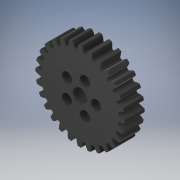
# Autodesk Inventor part: SE04
Saved by Autodesk Inventor 2017 SP1 (Build 210196100, 196)
## iProperties
Created: 2019-09-08
Part Number: SE04
Material: ABS Plastic
Document SubType Name: Modeling
Designer: Zach
Density: 1.06 g/cm^3
Appearance: Smooth - Black
Author: Zach
Autodesk Inventor part; units mm, degrees
(part 1 of 3)
ref_plane "YZ Plane" through (0, 0, 0) normal (1, 0, 0) x (0, 1, 0)
ref_plane "XZ Plane" through (0, 0, 0) normal (0, 1, 0) x (-1, 0, 0)
ref_plane "XY Plane" through (0, 0, 0) normal (0, 0, 1) x (1, 0, 0)
sketch "Sketch1" plane through (0, 0, 0) normal (0, 0, 1) x (1, 0, 0)
  arc A0 (-5.932911, 18.328081) -> (-5.539067, 18.99752) centre (-6.113075, 18.884647) ccw
  arc A1 (-5.932911, 18.328081) -> (-6.374085, 18.179357) centre (0.000012, -0.000078) ccw
  arc A2 (-7.092838, 18.47373) -> (-6.374085, 18.179357) centre (-6.567646, 18.731407) ccw
  spline S0 degree 3 poles (-9.030081, 20.608353) (-9.030081, 20.608353) (-9.030081, 20.608353) (-9.030081, 20.608353) (-9.030081, 20.608353) (-9.030081, 20.608353) (-9.030081, 20.608353) (-9.030081, 20.608353) (-9.030081, 20.608353) (-9.030081, 20.608353) (-9.030081, 20.608353) (-9.030081, 20.608353) (-9.030081, 20.608353) (-9.030081, 20.608353) (-9.030081, 20.608353) (-9.030029, 20.608313) (-9.023051, 20.602936) (-9.001036, 20.585861) (-8.989622, 20.576988) (-8.960537, 20.554257) (-8.942361, 20.539987) (-8.89306, 20.500976) (-8.860016, 20.474587) (-8.784661, 20.413566) (-8.741901, 20.378438) (-8.699366, 20.342893) knots 0 0 0 0 0.00003245 0.00003245 0.0000697 0.0000697 0.00012943 0.00012943 0.00021582 0.00021582 0.0003445 0.0003445 0.00053795 0.00053795 0.00077231 0.00077231 0.2100469 0.2100469 0.34914837 0.34914837 0.50737768 0.50737768 0.73605088 0.73605088 1 1 1 1
  spline S1 degree 3 poles (-8.699366, 20.342893) (-8.656399, 20.306988) (-8.538521, 20.206837) (-8.349354, 20.038244) (-8.135582, 19.833364) (-7.929716, 19.620545) (-7.73211, 19.400023) (-7.543618, 19.171666) (-7.362724, 18.937364) (-7.208648, 18.70567) (-7.128209, 18.545822) (-7.092838, 18.47373) knots 0 0 0 0 0.06771151 0.18704119 0.30636988 0.42569807 0.54502619 0.66435448 0.78368001 0.9029743 1 1 1 1
  arc A3 (-9.030081, 20.608353) -> (-10.023313, 20.143977) centre (0.000012, -0.000078) ccw
  arc A4 (-8.699366, 20.342893) -> (-10.031681, 19.719982) centre (0.000012, -0.000078) ccw
  arc A5 (-8.699366, 20.342893) -> (-10.031681, 19.719982) centre (0.000012, -0.000078) ccw
  spline S2 degree 3 poles (-10.031681, 19.719982) (-10.031681, 19.75177) (-10.031532, 19.78354) (-10.030954, 19.847219) (-10.030514, 19.879031) (-10.029214, 19.951703) (-10.028259, 19.991016) (-10.02666, 20.04753) (-10.026026, 20.067566) (-10.024905, 20.101012) (-10.02442, 20.114464) (-10.023579, 20.137231) (-10.023315, 20.14392) (-10.023313, 20.143977) (-10.023313, 20.143977) (-10.023313, 20.143977) (-10.023313, 20.143977) (-10.023313, 20.143977) (-10.023313, 20.143977) (-10.023313, 20.143977) (-10.023313, 20.143977) (-10.023313, 20.143977) (-10.023313, 20.143977) (-10.023313, 20.143977) (-10.023313, 20.143977) (-10.023313, 20.143977) (-10.023313, 20.143977) (-10.023313, 20.143977) knots 0 0 0 0 0.15149146 0.15149146 0.30980507 0.30980507 0.53062052 0.53062052 0.67593445 0.67593445 0.81687728 0.81687728 0.99922753 0.99922753 0.99946194 0.99946194 0.99965543 0.99965543 0.99978413 0.99978413 0.99987055 0.99987055 0.99993028 0.99993028 0.99996754 0.99996754 1 1 1 1
  spline S3 degree 3 poles (-9.627554, 17.288649) (-9.660192, 17.362018) (-9.73127, 17.526243) (-9.81026, 17.793043) (-9.874055, 18.082094) (-9.928415, 18.373163) (-9.970919, 18.666201) (-10.002215, 18.960638) (-10.022351, 19.256051) (-10.030418, 19.509315) (-10.031681, 19.663988) (-10.031681, 19.719982) knots 0 0 0 0 0.0970257 0.21631999 0.33564552 0.45497381 0.57430193 0.69363012 0.81295881 0.93228849 1 1 1 1
  spline S4 degree 3 poles (-5.392039, 21.457821) (-5.384966, 21.488811) (-5.377751, 21.519752) (-5.363018, 21.581705) (-5.355509, 21.612623) (-5.338071, 21.683183) (-5.328393, 21.721297) (-5.314258, 21.776039) (-5.309181, 21.795432) (-5.300646, 21.82779) (-5.29718, 21.840797) (-5.292456, 21.858461) (-5.290962, 21.864015) (-5.290178, 21.86693) (-5.289963, 21.867728) (-5.289748, 21.868526) (-5.289533, 21.869324) knots 0 0 0 0 0.15652291 0.15652291 0.32009454 0.32009454 0.54824388 0.54824388 0.69838409 0.69838409 0.84400801 0.84400801 0.96647827 0.96647827 0.96647827 1 1 1 1
  arc A6 (-4.217871, 22.101041) -> (-5.289533, 21.869324) centre (0.000012, -0.000078) ccw
  arc A7 (-3.954517, 21.768646) -> (-5.392039, 21.457821) centre (0.000012, -0.000078) ccw
  arc A8 (-3.954517, 21.768646) -> (-5.392039, 21.457821) centre (0.000012, -0.000078) ccw
  spline S5 degree 3 poles (-4.217871, 22.101041) (-4.217871, 22.101041) (-4.217871, 22.101041) (-4.217871, 22.101041) (-4.217871, 22.101041) (-4.217871, 22.101041) (-4.217871, 22.101041) (-4.217871, 22.101041) (-4.217871, 22.101041) (-4.217871, 22.101041) (-4.217871, 22.101041) (-4.217871, 22.101041) (-4.21787, 22.101041) (-4.21787, 22.101041) (-4.21787, 22.101041) (-4.217829, 22.100991) (-4.212222, 22.094196) (-4.194559, 22.07265) (-4.185405, 22.06146) (-4.162108, 22.032827) (-4.147562, 22.01487) (-4.108178, 21.965866) (-4.081835, 21.932786) (-4.021948, 21.856527) (-3.988076, 21.812764) (-3.954517, 21.768646) knots 0 0 0 0 0.00003245 0.00003245 0.0000697 0.0000697 0.00012943 0.00012943 0.00021582 0.00021582 0.0003445 0.0003445 0.00053795 0.00053795 0.00077231 0.00077231 0.21004691 0.21004691 0.34914837 0.34914837 0.50737768 0.50737768 0.73605088 0.73605088 1 1 1 1
  spline S6 degree 3 poles (-4.217871, 22.101041) (-4.217871, 22.101041) (-4.217871, 22.101041) (-4.217871, 22.101041) (-4.217871, 22.101041) (-4.217871, 22.101041) (-4.217871, 22.101041) (-4.217871, 22.101041) (-4.217871, 22.101041) (-4.217871, 22.101041) (-4.217871, 22.101041) (-4.217871, 22.101041) (-4.21787, 22.101041) (-4.21787, 22.101041) (-4.21787, 22.101041) (-4.217829, 22.100991) (-4.212222, 22.094196) (-4.194559, 22.07265) (-4.185405, 22.06146) (-4.162108, 22.032827) (-4.147562, 22.01487) (-4.108178, 21.965866) (-4.081835, 21.932786) (-4.021948, 21.856527) (-3.988076, 21.812764) (-3.954517, 21.768646) knots 0 0 0 0 0.00003245 0.00003245 0.0000697 0.0000697 0.00012943 0.00012943 0.00021582 0.00021582 0.0003445 0.0003445 0.00053795 0.00053795 0.00077231 0.00077231 0.21004691 0.21004691 0.34914837 0.34914837 0.50737768 0.50737768 0.73605088 0.73605088 1 1 1 1
  spline S7 degree 3 poles (-5.539067, 18.99752) (-5.554561, 19.076312) (-5.587313, 19.252235) (-5.604954, 19.529923) (-5.60283, 19.825922) (-5.591058, 20.12179) (-5.567289, 20.416939) (-5.532282, 20.710959) (-5.486177, 21.003445) (-5.437686, 21.252154) (-5.404499, 21.403231) (-5.392039, 21.457821) knots 0 0 0 0 0.0970257 0.21631999 0.33564552 0.45497381 0.57430193 0.69363012 0.81295881 0.93228849 1 1 1 1
  spline S8 degree 3 poles (-3.954517, 21.768646) (-3.920617, 21.72408) (-3.82798, 21.600209) (-3.681072, 21.39375) (-3.51825, 21.146438) (-3.364902, 20.893145) (-3.221321, 20.634181) (-3.088369, 20.369606) (-2.964148, 20.100926) (-2.865491, 19.840755) (-2.822639, 19.667016) (-2.804197, 19.588861) knots 0 0 0 0 0.06771151 0.18704119 0.30636988 0.42569807 0.54502619 0.66435448 0.78368001 0.9029743 1 1 1 1
  arc A9 (-2.804197, 19.588861) -> (-2.168968, 19.141931) centre (-2.234833, 19.723211) ccw
  arc A10 (-1.705761, 19.188755) -> (-2.168968, 19.141931) centre (0.000012, -0.000078) ccw
  arc A11 (-1.705761, 19.188755) -> (-1.172828, 19.753771) centre (-1.75756, 19.771457) ccw
  spline S9 degree 3 poles (3.252223, 19.519482) (3.27245, 19.597194) (3.319271, 19.769907) (3.423862, 20.027749) (3.554205, 20.293513) (3.693183, 20.554973) (3.842659, 20.81058) (4.001769, 21.060294) (4.170213, 21.303811) (4.321813, 21.50685) (4.417263, 21.628566) (4.452175, 21.672344) knots 0 0 0 0 0.0970257 0.21631999 0.33564552 0.45497381 0.57430193 0.69363012 0.81295881 0.93228849 1 1 1 1
  arc A12 (2.606923, 19.087221) -> (3.252223, 19.519482) centre (2.686086, 19.66684) ccw
  arc A13 (2.606923, 19.087221) -> (2.14491, 19.144644) centre (0.000012, -0.000078) ccw
  arc A14 (1.625059, 19.72172) -> (2.14491, 19.144644) centre (2.210044, 19.726007) ccw
  spline S10 degree 3 poles (0.988628, 22.102824) (1.011761, 22.051832) (1.074512, 21.910453) (1.171795, 21.67648) (1.275503, 21.399138) (1.368643, 21.118072) (1.450999, 20.833651) (1.521744, 20.546125) (1.583064, 20.256539) (1.621354, 19.980939) (1.624471, 19.80202) (1.625059, 19.72172) knots 0 0 0 0 0.06771151 0.18704119 0.30636988 0.42569807 0.54502619 0.66435448 0.78368001 0.9029743 1 1 1 1
  arc A15 (0.988628, 22.102824) -> (-0.482018, 22.119671) centre (0.000012, -0.000078) ccw
  spline S11 degree 3 poles (-1.172828, 19.753771) (-1.1704, 19.834036) (-1.163185, 20.012837) (-1.118592, 20.287488) (-1.050655, 20.575593) (-0.973342, 20.861423) (-0.884491, 21.143883) (-0.784937, 21.422741) (-0.674904, 21.697635) (-0.572285, 21.929318) (-0.506312, 22.069222) (-0.482018, 22.119671) knots 0 0 0 0 0.0970257 0.21631999 0.33564552 0.45497381 0.57430193 0.69363012 0.81295881 0.93228849 1 1 1 1
  spline S12 degree 3 poles (-0.482018, 22.119671) (-0.468226, 22.14831) (-0.454306, 22.17687) (-0.426157, 22.233991) (-0.411957, 22.262463) (-0.379255, 22.327374) (-0.361338, 22.362379) (-0.335376, 22.412603) (-0.326112, 22.430379) (-0.31059, 22.460027) (-0.304316, 22.471937) (-0.29578, 22.488106) (-0.293088, 22.493189) (-0.291674, 22.495857) (-0.291288, 22.496587) (-0.290901, 22.497317) (-0.290514, 22.498047) knots 0 0 0 0 0.15652267 0.15652267 0.32009406 0.32009406 0.54824306 0.54824306 0.69838305 0.69838305 0.84400675 0.84400675 0.96647984 0.96647984 0.96647984 1 1 1 1
  arc A16 (0.805842, 22.485487) -> (-0.290514, 22.498047) centre (0.000012, -0.000078) ccw
  arc A17 (0.805842, 22.485487) -> (-0.290514, 22.498047) centre (0.000012, -0.000078) ccw
  arc A18 (0.988628, 22.102824) -> (-0.482018, 22.119671) centre (0.000012, -0.000078) ccw
  spline S13 degree 3 poles (0.805842, 22.485487) (0.805842, 22.485487) (0.805842, 22.485487) (0.805842, 22.485487) (0.805842, 22.485487) (0.805842, 22.485487) (0.805842, 22.485487) (0.805842, 22.485487) (0.805842, 22.485487) (0.805842, 22.485487) (0.805842, 22.485487) (0.805842, 22.485487) (0.805842, 22.485487) (0.805842, 22.485487) (0.805842, 22.485487) (0.805872, 22.485428) (0.809826, 22.477557) (0.822252, 22.452621) (0.828686, 22.439674) (0.845028, 22.406575) (0.855213, 22.385832) (0.882705, 22.329293) (0.901027, 22.29118) (0.942443, 22.203506) (0.965727, 22.153304) (0.988628, 22.102824) knots 0 0 0 0 0.00003245 0.00003245 0.0000697 0.0000697 0.00012942 0.00012942 0.00021582 0.00021582 0.0003445 0.0003445 0.00053794 0.00053794 0.00077231 0.00077231 0.2100469 0.2100469 0.34914836 0.34914836 0.50737768 0.50737768 0.73605088 0.73605088 1 1 1 1
  spline S14 degree 3 poles (5.882199, 21.32867) (5.893406, 21.273809) (5.923123, 21.122012) (5.965904, 20.872258) (6.005297, 20.578791) (6.033559, 20.284047) (6.050561, 19.988431) (6.055552, 19.692372) (6.050895, 19.396401) (6.026898, 19.119191) (5.990123, 18.944064) (5.972829, 18.865647) knots 0 0 0 0 0.06771151 0.18704119 0.30636988 0.42569807 0.54502619 0.66435448 0.78368001 0.9029743 1 1 1 1
  spline S15 degree 3 poles (5.789147, 21.742413) (5.789147, 21.742413) (5.789147, 21.742413) (5.789147, 21.742413) (5.789147, 21.742413) (5.789147, 21.742413) (5.789147, 21.742413) (5.789147, 21.742413) (5.789147, 21.742413) (5.789147, 21.742413) (5.789147, 21.742413) (5.789147, 21.742413) (5.789147, 21.742413) (5.789147, 21.742413) (5.789147, 21.742413) (5.789163, 21.742349) (5.791266, 21.733795) (5.797832, 21.706719) (5.801224, 21.692665) (5.809791, 21.656759) (5.815105, 21.63427) (5.829327, 21.573031) (5.838708, 21.531797) (5.859577, 21.437105) (5.871106, 21.382981) (5.882199, 21.32867) knots 0 0 0 0 0.00003245 0.00003245 0.0000697 0.0000697 0.00012943 0.00012943 0.00021582 0.00021582 0.0003445 0.0003445 0.00053795 0.00053795 0.00077231 0.00077231 0.2100469 0.2100469 0.34914837 0.34914837 0.50737768 0.50737768 0.73605088 0.73605088 1 1 1 1
  arc A19 (5.789147, 21.742413) -> (4.723074, 21.99862) centre (0.000012, -0.000078) ccw
  arc A20 (5.882199, 21.32867) -> (4.452175, 21.672344) centre (0.000012, -0.000078) ccw
  arc A21 (5.882199, 21.32867) -> (4.452175, 21.672344) centre (0.000012, -0.000078) ccw
  spline S16 degree 3 poles (4.452175, 21.672344) (4.471994, 21.697196) (4.491919, 21.721943) (4.532074, 21.771368) (4.552253, 21.795966) (4.598579, 21.851973) (4.623836, 21.882113) (4.660323, 21.925301) (4.673311, 21.94057) (4.695041, 21.966021) (4.703808, 21.976236) (4.715728, 21.990101) (4.719484, 21.994457) (4.721455, 21.996743) (4.721995, 21.997369) (4.722534, 21.997994) (4.723074, 21.99862) knots 0 0 0 0 0.15652248 0.15652248 0.32009367 0.32009367 0.54824239 0.54824239 0.69838219 0.69838219 0.84400572 0.84400572 0.96648113 0.96648113 0.96648113 1 1 1 1
  arc A22 (5.972829, 18.865647) -> (6.351234, 18.187361) centre (6.5441, 18.739654) ccw
  arc A23 (6.788886, 18.02857) -> (6.351234, 18.187361) centre (0.000012, -0.000078) ccw
  arc A24 (6.788886, 18.02857) -> (7.514194, 18.306401) centre (6.995042, 18.576042) ccw
  spline S17 degree 3 poles (9.163118, 20.138272) (9.187969, 20.158097) (9.2129, 20.177795) (9.263044, 20.217057) (9.28819, 20.236554) (9.345815, 20.280861) (9.377145, 20.304633) (9.422326, 20.338629) (9.438385, 20.350629) (9.465232, 20.370612) (9.476052, 20.378623) (9.494375, 20.392164) (9.499769, 20.39613) (9.499815, 20.396164) (9.499815, 20.396164) (9.499815, 20.396164) (9.499815, 20.396164) (9.499815, 20.396164) (9.499815, 20.396164) (9.499815, 20.396164) (9.499815, 20.396164) (9.499815, 20.396164) (9.499815, 20.396164) (9.499815, 20.396164) (9.499815, 20.396164) (9.499815, 20.396164) (9.499815, 20.396164) (9.499815, 20.396164) knots 0 0 0 0 0.15149146 0.15149146 0.30980507 0.30980507 0.53062052 0.53062052 0.67593445 0.67593445 0.81687728 0.81687728 0.99922753 0.99922753 0.99946194 0.99946194 0.99965543 0.99965543 0.99978413 0.99978413 0.99987054 0.99987054 0.99993028 0.99993028 0.99996754 0.99996754 1 1 1 1
  spline S18 degree 3 poles (7.514194, 18.306401) (7.551207, 18.377664) (7.635286, 18.535627) (7.794629, 18.763731) (7.980843, 18.993828) (8.174517, 19.217807) (8.377123, 19.433744) (8.58781, 19.641792) (8.806219, 19.841721) (8.999198, 20.005936) (9.11934, 20.10336) (9.163118, 20.138272) knots 0 0 0 0 0.0970257 0.21631999 0.33564552 0.45497381 0.57430193 0.69363012 0.81295881 0.93228849 1 1 1 1
  arc A25 (10.482149, 19.909158) -> (9.499815, 20.396164) centre (0, 0) ccw
  arc A26 (10.480814, 19.485004) -> (9.163118, 20.138272) centre (0.000012, -0.000078) ccw
  arc A27 (10.480814, 19.485004) -> (9.163118, 20.138272) centre (0.000012, -0.000078) ccw
  spline S19 degree 3 poles (10.482149, 19.909158) (10.482162, 19.908332) (10.482175, 19.907507) (10.482188, 19.906682) (10.482245, 19.902983) (10.482366, 19.89518) (10.482674, 19.872419) (10.482855, 19.85796) (10.483218, 19.821042) (10.483395, 19.797929) (10.483635, 19.735049) (10.483607, 19.692754) (10.482884, 19.595775) (10.482082, 19.540432) (10.480814, 19.485004) knots 0 0 0 0 0.03353252 0.03353252 0.03353252 0.18383499 0.18383499 0.32755206 0.32755206 0.49103168 0.49103168 0.72729262 0.72729262 1 1 1 1
  spline S20 degree 3 poles (10.480814, 19.485004) (10.479531, 19.429025) (10.474726, 19.274421) (10.460858, 19.021409) (10.433961, 18.726535) (10.395928, 18.432891) (10.346723, 18.140904) (10.285709, 17.851156) (10.215309, 17.563643) (10.130228, 17.298722) (10.055407, 17.136169) (10.021097, 17.063567) knots 0 0 0 0 0.06771151 0.18704119 0.30636988 0.42569807 0.54502619 0.66435448 0.78368001 0.9029743 1 1 1 1
  arc A28 (10.021097, 17.063567) -> (10.239082, 16.318084) centre (10.550009, 16.813614) ccw
  arc A29 (10.630426, 16.065888) -> (10.239082, 16.318084) centre (0.000012, -0.000078) ccw
  arc A30 (10.630426, 16.065888) -> (11.399372, 16.175357) centre (10.953237, 16.553759) ccw
  spline S21 degree 3 poles (14.553877, 16.664275) (14.54017, 16.609984) (14.501082, 16.460326) (14.431262, 16.216743) (14.339423, 15.935247) (14.237002, 15.657429) (14.124057, 15.383712) (14.000098, 15.114806) (13.867486, 14.850166) (13.725588, 14.61082) (13.616471, 14.468992) (13.566865, 14.405845) knots 0 0 0 0 0.06771151 0.18704119 0.30636988 0.42569807 0.54502619 0.66435448 0.78368001 0.9029743 1 1 1 1
  spline S22 degree 3 poles (14.649556, 17.077418) (14.649556, 17.077418) (14.649556, 17.077418) (14.649556, 17.077418) (14.649556, 17.077418) (14.649556, 17.077418) (14.649556, 17.077418) (14.649556, 17.077418) (14.649556, 17.077418) (14.649556, 17.077418) (14.649556, 17.077418) (14.649556, 17.077418) (14.649556, 17.077418) (14.649556, 17.077418) (14.649556, 17.077418) (14.649542, 17.077354) (14.647726, 17.068734) (14.641893, 17.041491) (14.638852, 17.027357) (14.630991, 16.99129) (14.626021, 16.968722) (14.612264, 16.907377) (14.602826, 16.866156) (14.580542, 16.771787) (14.567446, 16.71802) (14.553877, 16.664275) knots 0 0 0 0 0.00003245 0.00003245 0.0000697 0.0000697 0.00012943 0.00012943 0.00021582 0.00021582 0.0003445 0.0003445 0.00053795 0.00053795 0.00077231 0.00077231 0.2100469 0.2100469 0.34914837 0.34914837 0.50737768 0.50737768 0.73605088 0.73605088 1 1 1 1
  arc A31 (14.553877, 16.664275) -> (13.414584, 17.594379) centre (0.000012, -0.000078) ccw
  arc A32 (14.553877, 16.664275) -> (13.414584, 17.594379) centre (0.000012, -0.000078) ccw
  arc A33 (14.649556, 17.077418) -> (13.800221, 17.770804) centre (0.000012, -0.000078) ccw
  spline S23 degree 3 poles (13.414584, 17.594379) (13.443223, 17.608171) (13.471912, 17.621821) (13.529535, 17.64893) (13.558389, 17.662336) (13.624427, 17.692696) (13.660261, 17.708893) (13.711873, 17.731972) (13.730199, 17.740095) (13.760819, 17.753596) (13.77315, 17.758996) (13.789906, 17.766316) (13.79518, 17.768611) (13.797948, 17.769816) (13.798706, 17.770145) (13.799463, 17.770475) (13.800221, 17.770804) knots 0 0 0 0 0.15652247 0.15652247 0.32009365 0.32009365 0.54824235 0.54824235 0.69838214 0.69838214 0.84400566 0.84400566 0.96648121 0.96648121 0.96648121 1 1 1 1
  spline S24 degree 3 poles (11.399372, 16.175357) (11.451315, 16.236597) (11.568436, 16.37189) (11.774542, 16.558818) (12.007288, 16.741709) (12.245947, 16.916976) (12.491523, 17.082415) (12.743223, 17.238364) (13.000644, 17.38468) (13.225326, 17.501836) (13.364135, 17.570084) (13.414584, 17.594379) knots 0 0 0 0 0.0970257 0.21631999 0.33564552 0.45497381 0.57430193 0.69363012 0.81295881 0.93228849 1 1 1 1
  spline S25 degree 3 poles (14.712939, 13.233209) (14.777206, 13.281355) (14.921497, 13.387194) (15.164031, 13.523572) (15.431639, 13.650087) (15.703314, 13.767854) (15.979547, 13.874499) (16.259638, 13.970529) (16.543164, 14.055895) (16.788282, 14.120117) (16.938797, 14.155766) (16.993387, 14.168226) knots 0 0 0 0 0.0970257 0.21631999 0.33564552 0.45497381 0.57430193 0.69363012 0.81295881 0.93228849 1 1 1 1
  arc A34 (13.938913, 13.297591) -> (14.712939, 13.233209) centre (14.362192, 13.701398) ccw
  arc A35 (13.938913, 13.297591) -> (13.6135, 13.630547) centre (0.000012, -0.000078) ccw
  arc A36 (13.566865, 14.405845) -> (13.6135, 13.630547) centre (14.026897, 14.044464) ccw
  arc A37 (16.065978, -10.630492) -> (16.318174, -10.239147) centre (0.000012, -0.000078) ccw
  arc A38 (17.063657, -10.021162) -> (16.318174, -10.239147) centre (16.813703, -10.550075) ccw
  spline S26 degree 3 poles (19.485094, -10.480879) (19.429115, -10.479597) (19.27451, -10.474791) (19.021498, -10.460924) (18.726624, -10.434027) (18.432981, -10.395993) (18.140994, -10.346788) (17.851246, -10.285774) (17.563733, -10.215375) (17.298812, -10.130294) (17.136259, -10.055473) (17.063657, -10.021162) knots 0 0 0 0 0.06771151 0.18704119 0.30636988 0.42569807 0.54502619 0.66435448 0.78368001 0.9029743 1 1 1 1
  spline S27 degree 3 poles (19.90917, -10.482227) (19.908344, -10.48224) (19.907519, -10.482252) (19.906694, -10.482265) (19.902996, -10.482322) (19.895194, -10.482443) (19.872438, -10.482751) (19.857981, -10.482931) (19.82107, -10.483293) (19.797962, -10.483469) (19.735093, -10.483708) (19.692805, -10.483678) (19.595844, -10.482953) (19.540511, -10.482149) (19.485094, -10.480879) knots 0 0 0 0 0.03353318 0.03353318 0.03353318 0.18383447 0.18383447 0.32755164 0.32755164 0.49103136 0.49103136 0.72729245 0.72729245 1 1 1 1
  arc A39 (19.90917, -10.482227) -> (20.396176, -9.499893) centre (0.000012, -0.000078) ccw
  arc A40 (19.485094, -10.480879) -> (20.138362, -9.163183) centre (0.000012, -0.000078) ccw
  arc A41 (19.485094, -10.480879) -> (20.138362, -9.163183) centre (0.000012, -0.000078) ccw
  spline S28 degree 3 poles (20.138362, -9.163183) (20.158181, -9.188036) (20.177873, -9.212968) (20.217124, -9.263114) (20.236615, -9.288261) (20.280908, -9.345888) (20.304673, -9.377219) (20.338659, -9.422401) (20.350655, -9.438461) (20.370632, -9.465309) (20.37864, -9.476129) (20.392177, -9.494453) (20.396142, -9.499847) (20.396176, -9.499893) (20.396176, -9.499893) (20.396176, -9.499893) (20.396176, -9.499893) (20.396176, -9.499893) (20.396176, -9.499893) (20.396176, -9.499893) (20.396176, -9.499893) (20.396176, -9.499893) (20.396176, -9.499893) (20.396176, -9.499893) (20.396176, -9.499893) (20.396176, -9.499893) (20.396176, -9.499893) (20.396176, -9.499893) knots 0 0 0 0 0.15149146 0.15149146 0.30980507 0.30980507 0.53062052 0.53062052 0.67593445 0.67593445 0.81687728 0.81687728 0.99922753 0.99922753 0.99946194 0.99946194 0.99965543 0.99965543 0.99978413 0.99978413 0.99987055 0.99987055 0.99993028 0.99993028 0.99996754 0.99996754 1 1 1 1
  spline S29 degree 3 poles (16.993387, 14.168226) (17.024378, 14.175299) (17.055385, 14.182223) (17.117595, 14.19583) (17.148708, 14.20248) (17.219847, 14.217384) (17.258387, 14.225201) (17.31384, 14.236217) (17.333515, 14.240057) (17.366371, 14.246407) (17.379595, 14.248927) (17.401977, 14.253173) (17.408557, 14.254405) (17.408614, 14.254416) (17.408614, 14.254416) (17.408614, 14.254416) (17.408614, 14.254416) (17.408614, 14.254416) (17.408614, 14.254416) (17.408614, 14.254416) (17.408614, 14.254416) (17.408614, 14.254416) (17.408614, 14.254416) (17.408614, 14.254416) (17.408614, 14.254416) (17.408614, 14.254416) (17.408614, 14.254416) (17.408614, 14.254416) knots 0 0 0 0 0.15149146 0.15149146 0.30980507 0.30980507 0.53062052 0.53062052 0.67593445 0.67593445 0.81687728 0.81687728 0.99922753 0.99922753 0.99946194 0.99946194 0.99965543 0.99965543 0.99978413 0.99978413 0.99987054 0.99987054 0.99993028 0.99993028 0.99996754 0.99996754 1 1 1 1
  arc A42 (17.897148, 13.007925) -> (16.993387, 14.168226) centre (0.000012, -0.000078) ccw
  arc A43 (17.897148, 13.007925) -> (16.993387, 14.168226) centre (0.000012, -0.000078) ccw
  arc A44 (18.082362, 13.389419) -> (17.408614, 14.254416) centre (0.000012, -0.000078) ccw
  spline S30 degree 3 poles (18.082362, 13.389419) (18.082362, 13.389419) (18.082362, 13.389419) (18.082362, 13.389419) (18.082362, 13.389419) (18.082362, 13.389419) (18.082362, 13.389419) (18.082362, 13.389419) (18.082362, 13.389419) (18.082362, 13.389419) (18.082362, 13.389419) (18.082362, 13.389419) (18.082362, 13.389419) (18.082362, 13.389419) (18.082361, 13.389419) (18.082334, 13.38936) (18.078645, 13.38136) (18.066896, 13.356098) (18.060786, 13.342995) (18.045097, 13.309582) (18.03523, 13.288686) (18.008167, 13.23194) (17.989793, 13.193852) (17.947069, 13.106808) (17.922337, 13.057303) (17.897148, 13.007925) knots 0 0 0 0 0.00003245 0.00003245 0.0000697 0.0000697 0.00012943 0.00012943 0.00021582 0.00021582 0.0003445 0.0003445 0.00053795 0.00053795 0.00077231 0.00077231 0.2100469 0.2100469 0.34914836 0.34914836 0.50737768 0.50737768 0.73605088 0.73605088 1 1 1 1
  arc A45 (16.432335, 11.025749) -> (16.30528, 10.259512) centre (16.800418, 10.571063) ccw
  arc A46 (16.548445, 9.862494) -> (16.30528, 10.259512) centre (0.000012, -0.000078) ccw
  spline S31 degree 3 poles (17.897148, 13.007925) (17.871704, 12.958046) (17.800294, 12.820837) (17.678023, 12.598898) (17.525848, 12.344896) (17.364174, 12.096835) (17.193153, 11.855112) (17.012465, 11.620532) (16.824289, 11.392037) (16.63269, 11.190266) (16.494749, 11.076275) (16.432335, 11.025749) knots 0 0 0 0 0.06771151 0.18704119 0.30636988 0.42569807 0.54502619 0.66435448 0.78368001 0.9029743 1 1 1 1
  arc A47 (16.548445, 9.862494) -> (17.288739, 9.627488) centre (17.050967, 10.161988) ccw
  spline S32 degree 3 poles (17.288739, 9.627488) (17.362108, 9.660126) (17.526333, 9.731205) (17.793133, 9.810194) (18.082183, 9.873989) (18.373252, 9.92835) (18.66629, 9.970853) (18.960728, 10.00215) (19.256141, 10.022285) (19.509404, 10.030353) (19.664078, 10.031615) (19.720072, 10.031615) knots 0 0 0 0 0.0970257 0.21631999 0.33564552 0.45497381 0.57430193 0.69363012 0.81295881 0.93228849 1 1 1 1
  arc A48 (18.082362, 13.389419) -> (17.408614, 14.254416) centre (0.000012, -0.000078) ccw
  spline S33 degree 3 poles (18.997609, 5.539001) (19.076402, 5.554495) (19.252325, 5.587248) (19.530013, 5.604888) (19.826012, 5.602764) (20.12188, 5.590993) (20.417028, 5.567223) (20.711048, 5.532217) (21.003535, 5.486112) (21.252244, 5.437621) (21.40332, 5.404433) (21.457911, 5.391973) knots 0 0 0 0 0.0970257 0.21631999 0.33564552 0.45497381 0.57430193 0.69363012 0.81295881 0.93228849 1 1 1 1
  arc A49 (18.32817, 5.932845) -> (18.997609, 5.539001) centre (18.884737, 6.113009) ccw
  arc A50 (18.32817, 5.932845) -> (18.179447, 6.374019) centre (0.000012, -0.000078) ccw
  arc A51 (18.47382, 7.092773) -> (18.179447, 6.374019) centre (18.731497, 6.56758) ccw
  spline S34 degree 3 poles (20.342983, 8.6993) (20.307077, 8.656333) (20.206926, 8.538455) (20.038334, 8.349288) (19.833454, 8.135517) (19.620634, 7.92965) (19.400113, 7.732044) (19.171756, 7.543552) (18.937454, 7.362659) (18.70576, 7.208582) (18.545911, 7.128143) (18.47382, 7.092773) knots 0 0 0 0 0.06771151 0.18704119 0.30636988 0.42569807 0.54502619 0.66435448 0.78368001 0.9029743 1 1 1 1
  spline S35 degree 3 poles (20.608443, 9.030015) (20.608443, 9.030015) (20.608443, 9.030015) (20.608443, 9.030015) (20.608443, 9.030015) (20.608443, 9.030015) (20.608443, 9.030015) (20.608443, 9.030015) (20.608443, 9.030015) (20.608443, 9.030015) (20.608443, 9.030015) (20.608443, 9.030015) (20.608443, 9.030015) (20.608443, 9.030015) (20.608443, 9.030015) (20.608402, 9.029963) (20.603026, 9.022986) (20.585951, 9.000971) (20.577078, 8.989556) (20.554347, 8.960471) (20.540077, 8.942295) (20.501066, 8.892994) (20.474677, 8.85995) (20.413655, 8.784595) (20.378527, 8.741835) (20.342983, 8.6993) knots 0 0 0 0 0.00003245 0.00003245 0.0000697 0.0000697 0.00012943 0.00012943 0.00021582 0.00021582 0.0003445 0.0003445 0.00053795 0.00053795 0.00077231 0.00077231 0.2100469 0.2100469 0.34914837 0.34914837 0.50737768 0.50737768 0.73605088 0.73605088 1 1 1 1
  spline S36 degree 3 poles (19.720072, 10.031615) (19.751859, 10.031615) (19.78363, 10.031466) (19.847308, 10.030888) (19.879121, 10.030448) (19.951793, 10.029148) (19.991105, 10.028194) (20.04762, 10.026594) (20.067656, 10.02596) (20.101102, 10.024839) (20.114554, 10.024354) (20.132827, 10.023679) (20.138574, 10.023459) (20.141591, 10.023343) (20.142416, 10.023311) (20.143242, 10.023279) (20.144067, 10.023247) knots 0 0 0 0 0.15652247 0.15652247 0.32009364 0.32009364 0.54824234 0.54824234 0.69838213 0.69838213 0.84400565 0.84400565 0.96648122 0.96648122 0.96648122 1 1 1 1
  arc A52 (20.342983, 8.6993) -> (19.720072, 10.031615) centre (0.000012, -0.000078) ccw
  arc A53 (20.342983, 8.6993) -> (19.720072, 10.031615) centre (0.000012, -0.000078) ccw
  arc A54 (20.608443, 9.030015) -> (20.144067, 10.023247) centre (0.000012, -0.000078) ccw
  arc A55 (21.742503, -5.789213) -> (21.998709, -4.723139) centre (0.000012, -0.000078) ccw
  arc A56 (21.32876, -5.882265) -> (21.672434, -4.452241) centre (0.000012, -0.000078) ccw
  arc A57 (21.32876, -5.882265) -> (21.672434, -4.452241) centre (0.000012, -0.000078) ccw
  spline S37 degree 3 poles (21.742503, -5.789213) (21.741701, -5.789409) (21.7409, -5.789605) (21.740098, -5.789801) (21.736506, -5.79068) (21.728926, -5.792534) (21.706809, -5.797897) (21.692755, -5.80129) (21.656849, -5.809856) (21.63436, -5.81517) (21.573121, -5.829392) (21.531887, -5.838774) (21.437195, -5.859642) (21.38307, -5.871172) (21.32876, -5.882265) knots 0 0 0 0 0.03353253 0.03353253 0.03353253 0.18383498 0.18383498 0.32755205 0.32755205 0.49103167 0.49103167 0.72729262 0.72729262 1 1 1 1
  arc A58 (18.865736, -5.972895) -> (18.187451, -6.3513) centre (18.739744, -6.544166) ccw
  arc A59 (18.02866, -6.788951) -> (18.187451, -6.3513) centre (0.000012, -0.000078) ccw
  arc A60 (18.02866, -6.788951) -> (18.306491, -7.514259) centre (18.576131, -6.995107) ccw
  spline S38 degree 3 poles (18.306491, -7.514259) (18.377753, -7.551272) (18.535717, -7.635352) (18.763821, -7.794695) (18.993918, -7.980909) (19.217897, -8.174582) (19.433834, -8.377188) (19.641881, -8.587876) (19.841811, -8.806284) (20.006025, -8.999264) (20.10345, -9.119405) (20.138362, -9.163183) knots 0 0 0 0 0.0970257 0.21631999 0.33564552 0.45497381 0.57430193 0.69363012 0.81295881 0.93228849 1 1 1 1
  spline S39 degree 3 poles (21.32876, -5.882265) (21.273899, -5.893471) (21.122102, -5.923189) (20.872347, -5.96597) (20.578881, -6.005363) (20.284137, -6.033625) (19.988521, -6.050627) (19.692461, -6.055617) (19.396491, -6.05096) (19.11928, -6.026963) (18.944153, -5.990189) (18.865736, -5.972895) knots 0 0 0 0 0.06771151 0.18704119 0.30636988 0.42569807 0.54502619 0.66435448 0.78368001 0.9029743 1 1 1 1
  spline S40 degree 3 poles (21.457911, 5.391973) (21.488901, 5.3849) (21.519842, 5.377685) (21.581795, 5.362952) (21.612712, 5.355444) (21.683273, 5.338006) (21.721387, 5.328327) (21.776129, 5.314192) (21.795521, 5.309116) (21.827879, 5.300581) (21.840887, 5.297114) (21.862895, 5.291228) (21.869358, 5.289483) (21.869413, 5.289468) (21.869413, 5.289468) (21.869413, 5.289468) (21.869413, 5.289468) (21.869413, 5.289468) (21.869413, 5.289468) (21.869413, 5.289468) (21.869413, 5.289468) (21.869413, 5.289468) (21.869413, 5.289468) (21.869413, 5.289468) (21.869413, 5.289468) (21.869413, 5.289468) (21.869413, 5.289468) (21.869413, 5.289468) knots 0 0 0 0 0.15149146 0.15149146 0.30980507 0.30980507 0.53062052 0.53062052 0.67593445 0.67593445 0.81687728 0.81687728 0.99922753 0.99922753 0.99946194 0.99946194 0.99965543 0.99965543 0.99978414 0.99978414 0.99987055 0.99987055 0.99993029 0.99993029 0.99996754 0.99996754 1 1 1 1
  arc A61 (21.768736, 3.954452) -> (21.457911, 5.391973) centre (0.000012, -0.000078) ccw
  arc A62 (21.768736, 3.954452) -> (21.457911, 5.391973) centre (0.000012, -0.000078) ccw
  arc A63 (22.101131, 4.217805) -> (21.869413, 5.289468) centre (0.000012, -0.000078) ccw
  spline S41 degree 3 poles (22.101131, 4.217805) (22.101131, 4.217805) (22.101131, 4.217805) (22.101131, 4.217805) (22.101131, 4.217805) (22.101131, 4.217805) (22.101131, 4.217805) (22.101131, 4.217805) (22.101131, 4.217805) (22.101131, 4.217805) (22.101131, 4.217805) (22.101131, 4.217805) (22.101131, 4.217805) (22.101131, 4.217805) (22.101131, 4.217805) (22.10108, 4.217763) (22.094286, 4.212157) (22.07274, 4.194493) (22.06155, 4.185339) (22.032917, 4.162042) (22.01496, 4.147497) (21.965956, 4.108112) (21.932876, 4.081769) (21.856616, 4.021882) (21.812854, 3.988011) (21.768736, 3.954452) knots 0 0 0 0 0.00003245 0.00003245 0.0000697 0.0000697 0.00012943 0.00012943 0.00021582 0.00021582 0.0003445 0.0003445 0.00053795 0.00053795 0.00077231 0.00077231 0.21004691 0.21004691 0.34914837 0.34914837 0.50737768 0.50737768 0.73605088 0.73605088 1 1 1 1
  spline S42 degree 3 poles (21.768736, 3.954452) (21.724169, 3.920552) (21.600299, 3.827915) (21.39384, 3.681006) (21.146528, 3.518184) (20.893235, 3.364836) (20.634271, 3.221255) (20.369696, 3.088303) (20.101015, 2.964082) (19.840845, 2.865426) (19.667105, 2.822573) (19.588951, 2.804131) knots 0 0 0 0 0.06771151 0.18704119 0.30636988 0.42569807 0.54502619 0.66435448 0.78368001 0.9029743 1 1 1 1
  arc A64 (19.188845, 1.705696) -> (19.14202, 2.168903) centre (0.000012, -0.000078) ccw
  arc A65 (19.188845, 1.705696) -> (19.753861, 1.172762) centre (19.771547, 1.757495) ccw
  spline S43 degree 3 poles (19.753861, 1.172762) (19.834125, 1.170334) (20.012926, 1.163119) (20.287577, 1.118526) (20.575682, 1.050589) (20.861513, 0.973276) (21.143972, 0.884426) (21.422831, 0.784871) (21.697725, 0.674838) (21.929408, 0.57222) (22.069312, 0.506247) (22.11976, 0.481952) knots 0 0 0 0 0.0970257 0.21631999 0.33564552 0.45497381 0.57430193 0.69363012 0.81295881 0.93228849 1 1 1 1
  arc A66 (19.588951, 2.804131) -> (19.14202, 2.168903) centre (19.723301, 2.234768) ccw
  spline S44 degree 3 poles (19.519572, -3.252288) (19.597284, -3.272516) (19.769996, -3.319337) (20.027838, -3.423928) (20.293603, -3.554271) (20.555063, -3.693249) (20.81067, -3.842724) (21.060383, -4.001835) (21.303901, -4.170279) (21.50694, -4.321878) (21.628656, -4.417329) (21.672434, -4.452241) knots 0 0 0 0 0.0970257 0.21631999 0.33564552 0.45497381 0.57430193 0.69363012 0.81295881 0.93228849 1 1 1 1
  arc A67 (19.087311, -2.606988) -> (19.519572, -3.252288) centre (19.66693, -2.686152) ccw
  arc A68 (19.087311, -2.606988) -> (19.144734, -2.144976) centre (0.000012, -0.000078) ccw
  arc A69 (19.72181, -1.625125) -> (19.144734, -2.144976) centre (19.726097, -2.210109) ccw
  spline S45 degree 3 poles (22.102914, -0.988693) (22.051921, -1.011826) (21.910543, -1.074577) (21.67657, -1.171861) (21.399228, -1.275568) (21.118162, -1.368709) (20.833741, -1.451065) (20.546215, -1.52181) (20.256629, -1.58313) (19.981028, -1.621419) (19.802109, -1.624537) (19.72181, -1.625125) knots 0 0 0 0 0.06771151 0.18704119 0.30636988 0.42569807 0.54502619 0.66435448 0.78368001 0.9029743 1 1 1 1
  spline S46 degree 3 poles (22.485577, -0.805908) (22.484839, -0.806278) (22.484101, -0.806647) (22.483364, -0.807017) (22.480056, -0.808673) (22.47308, -0.812167) (22.45271, -0.822317) (22.439764, -0.828752) (22.406664, -0.845094) (22.385921, -0.855278) (22.329382, -0.882771) (22.29127, -0.901093) (22.203596, -0.942509) (22.153394, -0.965793) (22.102914, -0.988693) knots 0 0 0 0 0.03353406 0.03353406 0.03353406 0.18383379 0.18383379 0.32755107 0.32755107 0.49103093 0.49103093 0.72729222 0.72729222 1 1 1 1
  arc A70 (22.485577, -0.805908) -> (22.498136, 0.290448) centre (0.000012, -0.000078) ccw
  arc A71 (22.102914, -0.988693) -> (22.11976, 0.481952) centre (0.000012, -0.000078) ccw
  arc A72 (22.102914, -0.988693) -> (22.11976, 0.481952) centre (0.000012, -0.000078) ccw
  spline S47 degree 3 poles (22.11976, 0.481952) (22.1484, 0.46816) (22.17696, 0.454241) (22.234081, 0.426091) (22.262552, 0.411891) (22.327463, 0.379189) (22.362469, 0.361272) (22.412692, 0.335311) (22.430469, 0.326046) (22.460116, 0.310525) (22.472026, 0.304251) (22.488196, 0.295714) (22.493279, 0.293022) (22.495946, 0.291609) (22.496676, 0.291222) (22.497406, 0.290835) (22.498136, 0.290448) knots 0 0 0 0 0.15652292 0.15652292 0.32009458 0.32009458 0.54824394 0.54824394 0.69838416 0.69838416 0.8440081 0.8440081 0.96647816 0.96647816 0.96647816 1 1 1 1
  spline S48 degree 3 poles (21.672434, -4.452241) (21.697286, -4.47206) (21.722033, -4.491985) (21.771458, -4.532139) (21.796056, -4.552319) (21.852062, -4.598645) (21.882203, -4.623902) (21.925391, -4.660389) (21.94066, -4.673377) (21.96611, -4.695106) (21.976325, -4.703873) (21.99019, -4.715794) (21.994547, -4.71955) (21.996833, -4.721521) (21.997458, -4.72206) (21.998084, -4.7226) (21.998709, -4.723139) knots 0 0 0 0 0.1565225 0.1565225 0.32009372 0.32009372 0.54824247 0.54824247 0.69838228 0.69838228 0.84400583 0.84400583 0.96648099 0.96648099 0.96648099 1 1 1 1
  spline S49 degree 3 poles (-21.328736, 5.88211) (-21.273875, 5.893316) (-21.122078, 5.923034) (-20.872323, 5.965815) (-20.578857, 6.005207) (-20.284113, 6.033469) (-19.988497, 6.050471) (-19.692437, 6.055462) (-19.396467, 6.050805) (-19.119256, 6.026808) (-18.944129, 5.990034) (-18.865712, 5.972739) knots 0 0 0 0 0.06771151 0.18704119 0.30636988 0.42569807 0.54502619 0.66435448 0.78368001 0.9029743 1 1 1 1
  spline S50 degree 3 poles (-21.742479, 5.789058) (-21.741677, 5.789254) (-21.740876, 5.78945) (-21.740074, 5.789646) (-21.736482, 5.790525) (-21.728902, 5.792379) (-21.706785, 5.797742) (-21.692731, 5.801135) (-21.656825, 5.809701) (-21.634336, 5.815015) (-21.573097, 5.829237) (-21.531863, 5.838619) (-21.437171, 5.859487) (-21.383046, 5.871016) (-21.328736, 5.88211) knots 0 0 0 0 0.03353302 0.03353302 0.03353302 0.1838346 0.1838346 0.32755174 0.32755174 0.49103143 0.49103143 0.72729249 0.72729249 1 1 1 1
  arc A73 (-21.328736, 5.88211) -> (-21.67241, 4.452085) centre (0.000012, -0.000078) ccw
  arc A74 (-21.742479, 5.789058) -> (-21.998685, 4.722984) centre (0.000012, -0.000078) ccw
  spline S51 degree 3 poles (-21.67241, 4.452085) (-21.697262, 4.471904) (-21.722008, 4.49183) (-21.771434, 4.531984) (-21.796032, 4.552163) (-21.852038, 4.59849) (-21.882179, 4.623747) (-21.925366, 4.660234) (-21.940636, 4.673221) (-21.966086, 4.694951) (-21.976301, 4.703718) (-21.990166, 4.715638) (-21.994522, 4.719394) (-21.996808, 4.721365) (-21.997434, 4.721905) (-21.99806, 4.722444) (-21.998685, 4.722984) knots 0 0 0 0 0.15652271 0.15652271 0.32009414 0.32009414 0.54824319 0.54824319 0.69838321 0.69838321 0.84400695 0.84400695 0.9664796 0.9664796 0.9664796 1 1 1 1
  arc A75 (-21.328736, 5.88211) -> (-21.67241, 4.452085) centre (0.000012, -0.000078) ccw
  arc A76 (-19.588926, -2.804287) -> (-19.141996, -2.169058) centre (-19.723277, -2.234923) ccw
  spline S52 degree 3 poles (-21.768711, -3.954607) (-21.724145, -3.920707) (-21.600275, -3.82807) (-21.393816, -3.681161) (-21.146504, -3.51834) (-20.893211, -3.364992) (-20.634247, -3.22141) (-20.369672, -3.088459) (-20.100991, -2.964238) (-19.840821, -2.865581) (-19.667081, -2.822729) (-19.588926, -2.804287) knots 0 0 0 0 0.06771151 0.18704119 0.30636988 0.42569807 0.54502619 0.66435448 0.78368001 0.9029743 1 1 1 1
  spline S53 degree 3 poles (-22.101107, -4.21796) (-22.101107, -4.21796) (-22.101107, -4.21796) (-22.101107, -4.21796) (-22.101107, -4.21796) (-22.101107, -4.21796) (-22.101107, -4.21796) (-22.101107, -4.21796) (-22.101107, -4.21796) (-22.101107, -4.21796) (-22.101107, -4.21796) (-22.101107, -4.21796) (-22.101107, -4.21796) (-22.101107, -4.21796) (-22.101107, -4.21796) (-22.101056, -4.217918) (-22.094262, -4.212312) (-22.072716, -4.194649) (-22.061525, -4.185494) (-22.032893, -4.162197) (-22.014936, -4.147652) (-21.965932, -4.108268) (-21.932852, -4.081924) (-21.856592, -4.022037) (-21.81283, -3.988166) (-21.768711, -3.954607) knots 0 0 0 0 0.00003245 0.00003245 0.0000697 0.0000697 0.00012942 0.00012942 0.00021582 0.00021582 0.0003445 0.0003445 0.00053795 0.00053795 0.00077231 0.00077231 0.2100469 0.2100469 0.34914836 0.34914836 0.50737768 0.50737768 0.73605088 0.73605088 1 1 1 1
  arc A77 (-22.101107, -4.21796) -> (-21.869389, -5.289623) centre (0.000012, -0.000078) ccw
  arc A78 (-21.768711, -3.954607) -> (-21.457887, -5.392129) centre (0.000012, -0.000078) ccw
  arc A79 (-21.768711, -3.954607) -> (-21.457887, -5.392129) centre (0.000012, -0.000078) ccw
  spline S54 degree 3 poles (-21.457887, -5.392129) (-21.488877, -5.385055) (-21.519818, -5.37784) (-21.581771, -5.363108) (-21.612688, -5.355599) (-21.683249, -5.338161) (-21.721363, -5.328483) (-21.776105, -5.314348) (-21.795497, -5.309271) (-21.827855, -5.300736) (-21.840862, -5.297269) (-21.862871, -5.291383) (-21.869334, -5.289638) (-21.869389, -5.289623) (-21.869389, -5.289623) (-21.869389, -5.289623) (-21.869389, -5.289623) (-21.869389, -5.289623) (-21.869389, -5.289623) (-21.869389, -5.289623) (-21.869389, -5.289623) (-21.869389, -5.289623) (-21.869389, -5.289623) (-21.869389, -5.289623) (-21.869389, -5.289623) (-21.869389, -5.289623) (-21.869389, -5.289623) (-21.869389, -5.289623) knots 0 0 0 0 0.15149146 0.15149146 0.30980507 0.30980507 0.53062052 0.53062052 0.67593445 0.67593445 0.81687728 0.81687728 0.99922753 0.99922753 0.99946194 0.99946194 0.99965543 0.99965543 0.99978414 0.99978414 0.99987055 0.99987055 0.99993029 0.99993029 0.99996754 0.99996754 1 1 1 1
  spline S55 degree 3 poles (-10.48079, -19.48516) (-10.479507, -19.42918) (-10.474702, -19.274576) (-10.460834, -19.021564) (-10.433937, -18.72669) (-10.395904, -18.433046) (-10.346699, -18.141059) (-10.285685, -17.851312) (-10.215285, -17.563798) (-10.130204, -17.298878) (-10.055383, -17.136325) (-10.021072, -17.063722) knots 0 0 0 0 0.06771151 0.18704119 0.30636988 0.42569807 0.54502619 0.66435448 0.78368001 0.9029743 1 1 1 1
  spline S56 degree 3 poles (-10.482137, -19.909235) (-10.482137, -19.909235) (-10.482137, -19.909235) (-10.482137, -19.909235) (-10.482137, -19.909235) (-10.482137, -19.909235) (-10.482137, -19.909235) (-10.482137, -19.909235) (-10.482137, -19.909235) (-10.482137, -19.909235) (-10.482137, -19.909235) (-10.482137, -19.909235) (-10.482137, -19.909235) (-10.482137, -19.909235) (-10.482137, -19.909235) (-10.482138, -19.909169) (-10.482285, -19.900362) (-10.482661, -19.872503) (-10.482841, -19.858047) (-10.483203, -19.821135) (-10.483379, -19.798027) (-10.483618, -19.735159) (-10.483589, -19.692871) (-10.482863, -19.59591) (-10.482059, -19.540577) (-10.48079, -19.48516) knots 0 0 0 0 0.00003245 0.00003245 0.0000697 0.0000697 0.00012943 0.00012943 0.00021582 0.00021582 0.0003445 0.0003445 0.00053795 0.00053795 0.00077231 0.00077231 0.2100469 0.2100469 0.34914837 0.34914837 0.50737768 0.50737768 0.73605088 0.73605088 1 1 1 1
  arc A80 (-10.48079, -19.48516) -> (-9.163094, -20.138427) centre (0.000012, -0.000078) ccw
  arc A81 (-10.48079, -19.48516) -> (-9.163094, -20.138427) centre (0.000012, -0.000078) ccw
  arc A82 (-10.482137, -19.909235) -> (-9.499803, -20.396242) centre (0.000012, -0.000078) ccw
  spline S57 degree 3 poles (-9.163094, -20.138427) (-9.187946, -20.158246) (-9.212878, -20.177938) (-9.263024, -20.21719) (-9.288171, -20.23668) (-9.345798, -20.280974) (-9.377129, -20.304739) (-9.422311, -20.338724) (-9.438371, -20.350721) (-9.465219, -20.370698) (-9.476039, -20.378706) (-9.494363, -20.392243) (-9.499757, -20.396208) (-9.499803, -20.396242) (-9.499803, -20.396242) (-9.499803, -20.396242) (-9.499803, -20.396242) (-9.499803, -20.396242) (-9.499803, -20.396242) (-9.499803, -20.396242) (-9.499803, -20.396242) (-9.499803, -20.396242) (-9.499803, -20.396242) (-9.499803, -20.396242) (-9.499803, -20.396242) (-9.499803, -20.396242) (-9.499803, -20.396242) (-9.499803, -20.396242) knots 0 0 0 0 0.15149146 0.15149146 0.30980507 0.30980507 0.53062052 0.53062052 0.67593445 0.67593445 0.81687728 0.81687728 0.99922753 0.99922753 0.99946194 0.99946194 0.99965543 0.99965543 0.99978413 0.99978413 0.99987055 0.99987055 0.99993028 0.99993028 0.99996754 0.99996754 1 1 1 1
  spline S58 degree 3 poles (-7.51417, -18.306557) (-7.551183, -18.377819) (-7.635262, -18.535783) (-7.794605, -18.763886) (-7.980819, -18.993983) (-8.174493, -19.217963) (-8.377098, -19.433899) (-8.587786, -19.641947) (-8.806195, -19.841876) (-8.999174, -20.006091) (-9.119316, -20.103515) (-9.163094, -20.138427) knots 0 0 0 0 0.0970257 0.21631999 0.33564552 0.45497381 0.57430193 0.69363012 0.81295881 0.93228849 1 1 1 1
  spline S59 degree 3 poles (-0.805818, -22.485643) (-0.806188, -22.484905) (-0.806557, -22.484167) (-0.806927, -22.483429) (-0.808583, -22.480122) (-0.812077, -22.473145) (-0.822228, -22.452776) (-0.828662, -22.439829) (-0.845004, -22.40673) (-0.855189, -22.385987) (-0.882681, -22.329448) (-0.901003, -22.291335) (-0.942419, -22.203661) (-0.965703, -22.153459) (-0.988604, -22.102979) knots 0 0 0 0 0.03353315 0.03353315 0.03353315 0.1838345 0.1838345 0.32755165 0.32755165 0.49103137 0.49103137 0.72729246 0.72729246 1 1 1 1
  arc A83 (-0.988604, -22.102979) -> (0.482042, -22.119826) centre (0.000012, -0.000078) ccw
  arc A84 (-0.988604, -22.102979) -> (0.482042, -22.119826) centre (0.000012, -0.000078) ccw
  arc A85 (-0.805818, -22.485643) -> (0.290538, -22.498202) centre (0.000012, -0.000078) ccw
  spline S60 degree 3 poles (0.482042, -22.119826) (0.46825, -22.148465) (0.45433, -22.177025) (0.426181, -22.234147) (0.411981, -22.262618) (0.379279, -22.327529) (0.361362, -22.362534) (0.3354, -22.412758) (0.326136, -22.430535) (0.310614, -22.460182) (0.30434, -22.472092) (0.293705, -22.492238) (0.290565, -22.498151) (0.290538, -22.498202) (0.290538, -22.498202) (0.290538, -22.498202) (0.290538, -22.498202) (0.290538, -22.498202) (0.290538, -22.498202) (0.290538, -22.498202) (0.290538, -22.498202) (0.290538, -22.498202) (0.290538, -22.498202) (0.290538, -22.498202) (0.290538, -22.498202) (0.290538, -22.498202) (0.290538, -22.498202) (0.290538, -22.498202) knots 0 0 0 0 0.15149146 0.15149146 0.30980507 0.30980507 0.53062052 0.53062052 0.67593445 0.67593445 0.81687728 0.81687728 0.99922753 0.99922753 0.99946194 0.99946194 0.99965543 0.99965543 0.99978413 0.99978413 0.99987055 0.99987055 0.99993028 0.99993028 0.99996754 0.99996754 1 1 1 1
  spline S61 degree 3 poles (17.594468, -13.414649) (17.60826, -13.443289) (17.621911, -13.471978) (17.649019, -13.529601) (17.662426, -13.558454) (17.692786, -13.624493) (17.708983, -13.660326) (17.732062, -13.711938) (17.740184, -13.730265) (17.753686, -13.760885) (17.759086, -13.773216) (17.766406, -13.789972) (17.768701, -13.795246) (17.769905, -13.798013) (17.770235, -13.798771) (17.770564, -13.799529) (17.770894, -13.800286) knots 0 0 0 0 0.15652274 0.15652274 0.32009419 0.32009419 0.54824328 0.54824328 0.69838332 0.69838332 0.84400708 0.84400708 0.96647943 0.96647943 0.96647943 1 1 1 1
  spline S62 degree 3 poles (16.175447, -11.399438) (16.236686, -11.45138) (16.37198, -11.568502) (16.558907, -11.774608) (16.741799, -12.007354) (16.917066, -12.246012) (17.082505, -12.491589) (17.238454, -12.743289) (17.38477, -13.00071) (17.501926, -13.225392) (17.570173, -13.3642) (17.594468, -13.414649) knots 0 0 0 0 0.0970257 0.21631999 0.33564552 0.45497381 0.57430193 0.69363012 0.81295881 0.93228849 1 1 1 1
  arc A86 (17.077508, -14.649622) -> (17.770894, -13.800286) centre (0.000012, -0.000078) ccw
  arc A87 (16.664365, -14.553942) -> (17.594468, -13.414649) centre (0.000012, -0.000078) ccw
  arc A88 (16.664365, -14.553942) -> (17.594468, -13.414649) centre (0.000012, -0.000078) ccw
  spline S63 degree 3 poles (17.077508, -14.649622) (17.077508, -14.649622) (17.077508, -14.649622) (17.077508, -14.649622) (17.077508, -14.649622) (17.077508, -14.649622) (17.077508, -14.649622) (17.077508, -14.649622) (17.077508, -14.649622) (17.077508, -14.649622) (17.077508, -14.649622) (17.077508, -14.649622) (17.077508, -14.649622) (17.077508, -14.649622) (17.077508, -14.649622) (17.077443, -14.649608) (17.068824, -14.647791) (17.04158, -14.641959) (17.027446, -14.638918) (16.99138, -14.631057) (16.968812, -14.626087) (16.907466, -14.61233) (16.866245, -14.602892) (16.771877, -14.580608) (16.71811, -14.567512) (16.664365, -14.553942) knots 0 0 0 0 0.00003245 0.00003245 0.0000697 0.0000697 0.00012943 0.00012943 0.00021582 0.00021582 0.0003445 0.0003445 0.00053795 0.00053795 0.00077231 0.00077231 0.2100469 0.2100469 0.34914836 0.34914836 0.50737768 0.50737768 0.73605088 0.73605088 1 1 1 1
  spline S64 degree 3 poles (16.664365, -14.553942) (16.610074, -14.540235) (16.460416, -14.501148) (16.216833, -14.431328) (15.935337, -14.339489) (15.657519, -14.237067) (15.383802, -14.124123) (15.114896, -14.000164) (14.850256, -13.867551) (14.61091, -13.725654) (14.469082, -13.616536) (14.405934, -13.566931) knots 0 0 0 0 0.06771151 0.18704119 0.30636988 0.42569807 0.54502619 0.66435448 0.78368001 0.9029743 1 1 1 1
  arc A89 (14.405934, -13.566931) -> (13.630636, -13.613565) centre (14.044554, -14.026962) ccw
  arc A90 (13.297681, -13.938979) -> (13.630636, -13.613565) centre (0.000012, -0.000078) ccw
  arc A91 (13.297681, -13.938979) -> (13.233298, -14.713005) centre (13.701488, -14.362258) ccw
  spline S65 degree 3 poles (14.168315, -16.993453) (14.175389, -17.024443) (14.182313, -17.05545) (14.19592, -17.117661) (14.202569, -17.148774) (14.217473, -17.219913) (14.225291, -17.258452) (14.236307, -17.313906) (14.240147, -17.33358) (14.246497, -17.366437) (14.249017, -17.37966) (14.253263, -17.402043) (14.254495, -17.408623) (14.254505, -17.408679) (14.254505, -17.408679) (14.254505, -17.408679) (14.254505, -17.408679) (14.254505, -17.408679) (14.254505, -17.408679) (14.254505, -17.408679) (14.254505, -17.408679) (14.254505, -17.40868) (14.254505, -17.40868) (14.254505, -17.40868) (14.254505, -17.40868) (14.254505, -17.40868) (14.254505, -17.40868) (14.254505, -17.40868) knots 0 0 0 0 0.15149146 0.15149146 0.30980507 0.30980507 0.53062052 0.53062052 0.67593445 0.67593445 0.81687728 0.81687728 0.99922753 0.99922753 0.99946194 0.99946194 0.99965543 0.99965543 0.99978414 0.99978414 0.99987055 0.99987055 0.99993028 0.99993028 0.99996754 0.99996754 1 1 1 1
  spline S66 degree 3 poles (13.233298, -14.713005) (13.281444, -14.777272) (13.387284, -14.921563) (13.523662, -15.164097) (13.650177, -15.431705) (13.767944, -15.70338) (13.874588, -15.979613) (13.970619, -16.259704) (14.055985, -16.54323) (14.120207, -16.788348) (14.155856, -16.938863) (14.168315, -16.993453) knots 0 0 0 0 0.0970257 0.21631999 0.33564552 0.45497381 0.57430193 0.69363012 0.81295881 0.93228849 1 1 1 1
  arc A92 (16.065978, -10.630492) -> (16.175447, -11.399438) centre (16.553849, -10.953303) ccw
  arc A93 (9.862583, -16.548511) -> (9.627578, -17.288804) centre (10.162077, -17.051033) ccw
  arc A94 (9.862583, -16.548511) -> (10.259602, -16.305346) centre (0.000012, -0.000078) ccw
  arc A95 (11.025839, -16.432401) -> (10.259602, -16.305346) centre (10.571152, -16.800484) ccw